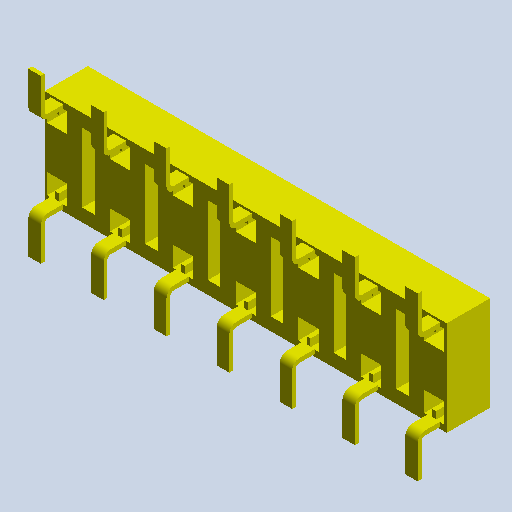
# Autodesk Inventor part: C-132-12-07-DV
Saved by Autodesk Inventor 2024.2 (Build 282272000, 272)
## iProperties
Category: PARTsolutions
Company: SAMTEC
Part Number: C-132-12-07-DV
Material: Generic
Catalog Web Link: www.cadenas.de
Description: C-132-Pins
Vendor: SAMTEC
Document SubType Name: Modeling
Designer: partserver
Manufacturer: SAMTEC
Mass: 0.0818982 g
Surface Area: 3.68105 cm^2
Volume: 0.0818982 cm^3
Density: 1 g/cm^3
Appearance: PSOLRGB-255-255-0
PSOL_IDENT_0: {$CADENAS_DATA\23d-libs\samtec\modelling\hle\parts\hle_pins.prj},176 {VTYP=3D},{NB=C-132-12-07-DV},{
PSOL_IDENT_1: LINA=C-132-12-07-DV},{NN=C-132},{DATE=08.04.2016 05:41:50},{GEOMDATE=08.04.2016 05:31:00},{VERSION=}
PSOL_IDENT_2: ,{LINEID=10},{WBVAR=POS,ESOPT},{WBNUMERIC=}  {NB=C-132-12-07-DV},{LINA=C-132-12-07-DV},{KT=DUMMY},{P
PSOL_IDENT_3: N=C-132-12-07-DV},{SERIES=HLE},{POSALG=  '02' , '-02' , '03' , '-03' , '04' , '-04' , '05' , '-05' ,
PSOL_IDENT_4: '06' , '-06' , '07' , '-07' , '08' , '-08' , '09' , '-09' , '10' , '-10' , '11' , '-11' , '12' , '-
PSOL_IDENT_5: 12' , '13' , '-13' , '14' , '-14' , '15' , '-15' , '16' , '-16' , '17' , '-17' , '18' , '-18' , '19'
PSOL_IDENT_6: , '-19' , '20' , '-20' , '21' , '-21' , '22' , '-22' , '23' , '-23' , '24' , '-24' , '25' , '-25' ,
PSOL_IDENT_7: '26' , '-26' , '27' , '-27' , '28' , '-28' , '29' , '-29' , '30' , '-30' , '31' , '-31' , '32' , '-
PSOL_IDENT_8: 32' , '33' , '-33' , '34' , '-34' , '35' , '-35' , '36' , '-36' , '37' , '-37' , '38' , '-38' , '39'
PSOL_IDENT_9: , '-39' , '40' , '-40'  , '41' , '-41' , '42' , '-42' , '43' , '-43' , '44' , '-44' , '45' , '-45'
PSOL_IDENT_10: , '46' , '-46' , '47' , '-47' , '48' , '-48' , '49' , '-49' , '50' , '-50'   , '51' , '-51' , '52' ,
PSOL_IDENT_11: '-52' , '53' , '-53' , '54' , '-54' , '55' , '-55' , '56' , '-56' , '57' , '-57' , '58' , '-58' , '
PSOL_IDENT_12: 59' , '-59' , '60' , '-60'  , '61' , '-61' , '62' , '-62' , '63' , '-63' , '64' , '-64' , '65' , '-6
PSOL_IDENT_13: 5' , '66' , '-66' , '67' , '-67' , '68' , '-68' , '69' , '-69' , '70' , '-70'  , '71' , '-71' , '72'
PSOL_IDENT_14: , '-72' , '73' , '-73' , '74' , '-74' , '75' , '-75'   },{POS=07},{LSALG=  '02' , '-02 - Surface Mo
PSOL_IDENT_15: unt'  },{LS=02},{ROPTALG=   'DV' , '-DV - Double Vertical'   },{ROPT=DV},{ESOPT=},{A=0.144},{B=0.138
PSOL_IDENT_16: },{L=0.700},{PINS=7},{H2=0.030},{W=0.2000},{PINH=0.025},{PINL=0.2590},{PINW=0.020},{PITCH=0.1000},{P
PSOL_IDENT_17: ITCH2=0.1000},{X=0.045},{ESOPTPN=}
NB: C-132-12-07-DV
NN: C-132
NT: Pins
NBSYN: $PN.
LINA: C-132-12-07-DV
CATALOG: Samtec
PN: C-132-12-07-DV
SERIES: HLE
POS: -07
LS: 02
ROPT: DV
ESOPT: Standard
A: 0.144
B: 0.138
L: 0.7
H2: 0.03
W: 0.2
PINH: 0.025
PINL: 0.259
PINW: 0.02
PITCH: 0.1
PITCH2: 0.1
X: 0.045
SUPPLIER: SAMTEC
ARTICLENO: C-132-12-07-DV
BOMINFO: C-132-12-07-DV
CREATOR: CADENAS GmbH
Title: C-132-12-07-DV
Author: Cadenas PARTsolutions
Comments: Pins
Autodesk Inventor part; units mm, degrees
sketch "Sketch_11" plane through (0, 2.5146, 0) normal (0, 1, 0) x (1, 0, 0)
  line L0 (-8.128, 1.9177) -> (-8.128, -1.9177)
  line L1 (-8.128, -1.9177) -> (8.128, -1.9177)
  line L2 (8.128, -1.9177) -> (8.128, 1.9177)
  line L3 (8.128, 1.9177) -> (-8.128, 1.9177)
  line L4 (7.2136, -0.8636) -> (7.2136, -1.6764)
  line L5 (7.2136, -1.6764) -> (7.5438, -1.6764)
  line L6 (7.5438, -1.6764) -> (7.5438, -1.3716)
  line L7 (7.5438, -1.3716) -> (7.6962, -1.3716)
  line L8 (7.6962, -1.3716) -> (7.6962, -1.6764)
  line L9 (7.6962, -1.6764) -> (8.0264, -1.6764)
  line L10 (8.0264, -1.6764) -> (8.0264, -0.8636)
  line L11 (8.0264, -0.8636) -> (7.2136, -0.8636)
  line L12 (7.2136, 0.8636) -> (8.0264, 0.8636)
  line L13 (8.0264, 0.8636) -> (8.0264, 1.6764)
  line L14 (8.0264, 1.6764) -> (7.6962, 1.6764)
  line L15 (7.6962, 1.6764) -> (7.6962, 1.3716)
  line L16 (7.6962, 1.3716) -> (7.5438, 1.3716)
  line L17 (7.5438, 1.3716) -> (7.5438, 1.6764)
  line L18 (7.5438, 1.6764) -> (7.2136, 1.6764)
  line L19 (7.2136, 1.6764) -> (7.2136, 0.8636)
  line L20 (6.096, 1.397) -> (6.096, -1.397)
  line L21 (6.096, -1.397) -> (6.604, -1.397)
  line L22 (6.604, -1.397) -> (6.604, 1.397)
  line L23 (6.604, 1.397) -> (6.096, 1.397)
  line L24 (4.6736, -0.8636) -> (4.6736, -1.6764)
  line L25 (4.6736, -1.6764) -> (5.0038, -1.6764)
  line L26 (5.0038, -1.6764) -> (5.0038, -1.3716)
  line L27 (5.0038, -1.3716) -> (5.1562, -1.3716)
  line L28 (5.1562, -1.3716) -> (5.1562, -1.6764)
  line L29 (5.1562, -1.6764) -> (5.4864, -1.6764)
  line L30 (5.4864, -1.6764) -> (5.4864, -0.8636)
  line L31 (5.4864, -0.8636) -> (4.6736, -0.8636)
  line L32 (4.6736, 0.8636) -> (5.4864, 0.8636)
  line L33 (5.4864, 0.8636) -> (5.4864, 1.6764)
  line L34 (5.4864, 1.6764) -> (5.1562, 1.6764)
  line L35 (5.1562, 1.6764) -> (5.1562, 1.3716)
  line L36 (5.1562, 1.3716) -> (5.0038, 1.3716)
  line L37 (5.0038, 1.3716) -> (5.0038, 1.6764)
  line L38 (5.0038, 1.6764) -> (4.6736, 1.6764)
  line L39 (4.6736, 1.6764) -> (4.6736, 0.8636)
  line L40 (3.556, 1.397) -> (3.556, -1.397)
  line L41 (3.556, -1.397) -> (4.064, -1.397)
  line L42 (4.064, -1.397) -> (4.064, 1.397)
  line L43 (4.064, 1.397) -> (3.556, 1.397)
  line L44 (2.1336, -0.8636) -> (2.1336, -1.6764)
  line L45 (2.1336, -1.6764) -> (2.4638, -1.6764)
  line L46 (2.4638, -1.6764) -> (2.4638, -1.3716)
  line L47 (2.4638, -1.3716) -> (2.6162, -1.3716)
  line L48 (2.6162, -1.3716) -> (2.6162, -1.6764)
  line L49 (2.6162, -1.6764) -> (2.9464, -1.6764)
  line L50 (2.9464, -1.6764) -> (2.9464, -0.8636)
  line L51 (2.9464, -0.8636) -> (2.1336, -0.8636)
  line L52 (2.1336, 0.8636) -> (2.9464, 0.8636)
  line L53 (2.9464, 0.8636) -> (2.9464, 1.6764)
  line L54 (2.9464, 1.6764) -> (2.6162, 1.6764)
  line L55 (2.6162, 1.6764) -> (2.6162, 1.3716)
  line L56 (2.6162, 1.3716) -> (2.4638, 1.3716)
  line L57 (2.4638, 1.3716) -> (2.4638, 1.6764)
  line L58 (2.4638, 1.6764) -> (2.1336, 1.6764)
  line L59 (2.1336, 1.6764) -> (2.1336, 0.8636)
  line L60 (1.016, 1.397) -> (1.016, -1.397)
  line L61 (1.016, -1.397) -> (1.524, -1.397)
  line L62 (1.524, -1.397) -> (1.524, 1.397)
  line L63 (1.524, 1.397) -> (1.016, 1.397)
  line L64 (-0.4064, -0.8636) -> (-0.4064, -1.6764)
  line L65 (-0.4064, -1.6764) -> (-0.0762, -1.6764)
  line L66 (-0.0762, -1.6764) -> (-0.0762, -1.3716)
  line L67 (-0.0762, -1.3716) -> (0.0762, -1.3716)
  line L68 (0.0762, -1.3716) -> (0.0762, -1.6764)
  line L69 (0.0762, -1.6764) -> (0.4064, -1.6764)
  line L70 (0.4064, -1.6764) -> (0.4064, -0.8636)
  line L71 (0.4064, -0.8636) -> (-0.4064, -0.8636)
  line L72 (-0.4064, 0.8636) -> (0.4064, 0.8636)
  line L73 (0.4064, 0.8636) -> (0.4064, 1.6764)
  line L74 (0.4064, 1.6764) -> (0.0762, 1.6764)
  line L75 (0.0762, 1.6764) -> (0.0762, 1.3716)
  line L76 (0.0762, 1.3716) -> (-0.0762, 1.3716)
  line L77 (-0.0762, 1.3716) -> (-0.0762, 1.6764)
  line L78 (-0.0762, 1.6764) -> (-0.4064, 1.6764)
  line L79 (-0.4064, 1.6764) -> (-0.4064, 0.8636)
  line L80 (-1.524, 1.397) -> (-1.524, -1.397)
  line L81 (-1.524, -1.397) -> (-1.016, -1.397)
  line L82 (-1.016, -1.397) -> (-1.016, 1.397)
  line L83 (-1.016, 1.397) -> (-1.524, 1.397)
  line L84 (-2.9464, -0.8636) -> (-2.9464, -1.6764)
  line L85 (-2.9464, -1.6764) -> (-2.6162, -1.6764)
  line L86 (-2.6162, -1.6764) -> (-2.6162, -1.3716)
  line L87 (-2.6162, -1.3716) -> (-2.4638, -1.3716)
  line L88 (-2.4638, -1.3716) -> (-2.4638, -1.6764)
  line L89 (-2.4638, -1.6764) -> (-2.1336, -1.6764)
  line L90 (-2.1336, -1.6764) -> (-2.1336, -0.8636)
  line L91 (-2.1336, -0.8636) -> (-2.9464, -0.8636)
  line L92 (-2.9464, 0.8636) -> (-2.1336, 0.8636)
  line L93 (-2.1336, 0.8636) -> (-2.1336, 1.6764)
  line L94 (-2.1336, 1.6764) -> (-2.4638, 1.6764)
  line L95 (-2.4638, 1.6764) -> (-2.4638, 1.3716)
  line L96 (-2.4638, 1.3716) -> (-2.6162, 1.3716)
  line L97 (-2.6162, 1.3716) -> (-2.6162, 1.6764)
  line L98 (-2.6162, 1.6764) -> (-2.9464, 1.6764)
  line L99 (-2.9464, 1.6764) -> (-2.9464, 0.8636)
  line L100 (-4.064, 1.397) -> (-4.064, -1.397)
  line L101 (-4.064, -1.397) -> (-3.556, -1.397)
  line L102 (-3.556, -1.397) -> (-3.556, 1.397)
  line L103 (-3.556, 1.397) -> (-4.064, 1.397)
  line L104 (-5.4864, -0.8636) -> (-5.4864, -1.6764)
  line L105 (-5.4864, -1.6764) -> (-5.1562, -1.6764)
  line L106 (-5.1562, -1.6764) -> (-5.1562, -1.3716)
  line L107 (-5.1562, -1.3716) -> (-5.0038, -1.3716)
  line L108 (-5.0038, -1.3716) -> (-5.0038, -1.6764)
  line L109 (-5.0038, -1.6764) -> (-4.6736, -1.6764)
  line L110 (-4.6736, -1.6764) -> (-4.6736, -0.8636)
  line L111 (-4.6736, -0.8636) -> (-5.4864, -0.8636)
  line L112 (-5.4864, 0.8636) -> (-4.6736, 0.8636)
  line L113 (-4.6736, 0.8636) -> (-4.6736, 1.6764)
  line L114 (-4.6736, 1.6764) -> (-5.0038, 1.6764)
  line L115 (-5.0038, 1.6764) -> (-5.0038, 1.3716)
  line L116 (-5.0038, 1.3716) -> (-5.1562, 1.3716)
  line L117 (-5.1562, 1.3716) -> (-5.1562, 1.6764)
  line L118 (-5.1562, 1.6764) -> (-5.4864, 1.6764)
  line L119 (-5.4864, 1.6764) -> (-5.4864, 0.8636)
  line L120 (-6.604, 1.397) -> (-6.604, -1.397)
  line L121 (-6.604, -1.397) -> (-6.096, -1.397)
  line L122 (-6.096, -1.397) -> (-6.096, 1.397)
  line L123 (-6.096, 1.397) -> (-6.604, 1.397)
  line L124 (-8.0264, -0.8636) -> (-8.0264, -1.6764)
  line L125 (-8.0264, -1.6764) -> (-7.6962, -1.6764)
  line L126 (-7.6962, -1.6764) -> (-7.6962, -1.3716)
  line L127 (-7.6962, -1.3716) -> (-7.5438, -1.3716)
  line L128 (-7.5438, -1.3716) -> (-7.5438, -1.6764)
  line L129 (-7.5438, -1.6764) -> (-7.2136, -1.6764)
  line L130 (-7.2136, -1.6764) -> (-7.2136, -0.8636)
  line L131 (-7.2136, -0.8636) -> (-8.0264, -0.8636)
  line L132 (-8.0264, 0.8636) -> (-7.2136, 0.8636)
  line L133 (-7.2136, 0.8636) -> (-7.2136, 1.6764)
  line L134 (-7.2136, 1.6764) -> (-7.5438, 1.6764)
  line L135 (-7.5438, 1.6764) -> (-7.5438, 1.3716)
  line L136 (-7.5438, 1.3716) -> (-7.6962, 1.3716)
  line L137 (-7.6962, 1.3716) -> (-7.6962, 1.6764)
  line L138 (-7.6962, 1.6764) -> (-8.0264, 1.6764)
  line L139 (-8.0264, 1.6764) -> (-8.0264, 0.8636)
  constraints: 280 end point
extrude "Extrusion1" add sketch "Sketch_11" against normal blind 1.7526
sketch "Sketch_12" plane through (0, 0, 0) normal (1, 0, 0) x (0, 1, 0)
  line L0 (-0.1524, 3.2893) -> (-0.1524, 1.9558)
  arc A0 (-0.1524, 1.9558) -> (0.1524, 1.651) centre (0.1524, 1.9558) ccw
  line L1 (0.1524, 1.651) -> (0.762, 1.651)
  line L2 (0.762, 1.651) -> (0.762, 1.8288)
  line L3 (0.762, 1.8288) -> (0.127, 1.8288)
  arc A1 (0, 1.9558) -> (0.127, 1.8288) centre (0.127, 1.9558) ccw
  line L4 (0, 1.9558) -> (0, 3.2893)
  line L5 (0, 3.2893) -> (-0.1524, 3.2893)
  constraints: 12 end point, 4 point on circle, 2 centre point
extrude "Extrusion2" add sketch "Sketch_12" along normal mid plane 16.256
sketch "Sketch_13" plane through (0, 0, 0) normal (1, 0, 0) x (0, 1, 0)
  arc A0 (0.1524, -1.651) -> (-0.1524, -1.9558) centre (0.1524, -1.9558) ccw
  line L0 (-0.1524, -1.9558) -> (-0.1524, -3.2893)
  line L1 (-0.1524, -3.2893) -> (0, -3.2893)
  line L2 (0, -3.2893) -> (0, -1.9558)
  arc A1 (0.127, -1.8288) -> (0, -1.9558) centre (0.127, -1.9558) ccw
  line L3 (0.127, -1.8288) -> (0.762, -1.8288)
  line L4 (0.762, -1.8288) -> (0.762, -1.651)
  line L5 (0.762, -1.651) -> (0.1524, -1.651)
  constraints: 12 end point, 4 point on circle, 2 centre point
extrude "Extrusion3" add sketch "Sketch_13" along normal mid plane 16.256
sketch "Sketch_5" plane through (0, 0, 0) normal (0, 0, 1) x (1, 0, 0)
  line L0 (-10.414, -3.556) -> (9.906, -3.556)
  line L1 (9.906, -3.556) -> (9.906, 0.762)
  line L2 (9.906, 0.762) -> (7.874, 0.762)
  line L3 (7.874, 0.762) -> (7.874, -3.048)
  line L4 (7.874, -3.048) -> (7.366, -3.048)
  line L5 (7.366, -3.048) -> (7.366, 0.762)
  line L6 (7.366, 0.762) -> (5.334, 0.762)
  line L7 (5.334, 0.762) -> (5.334, -3.048)
  line L8 (5.334, -3.048) -> (4.826, -3.048)
  line L9 (4.826, -3.048) -> (4.826, 0.762)
  line L10 (4.826, 0.762) -> (2.794, 0.762)
  line L11 (2.794, 0.762) -> (2.794, -3.048)
  line L12 (2.794, -3.048) -> (2.286, -3.048)
  line L13 (2.286, -3.048) -> (2.286, 0.762)
  line L14 (2.286, 0.762) -> (0.254, 0.762)
  line L15 (0.254, 0.762) -> (0.254, -3.048)
  line L16 (0.254, -3.048) -> (-0.254, -3.048)
  line L17 (-0.254, -3.048) -> (-0.254, 0.762)
  line L18 (-0.254, 0.762) -> (-2.286, 0.762)
  line L19 (-2.286, 0.762) -> (-2.286, -3.048)
  line L20 (-2.286, -3.048) -> (-2.794, -3.048)
  line L21 (-2.794, -3.048) -> (-2.794, 0.762)
  line L22 (-2.794, 0.762) -> (-4.826, 0.762)
  line L23 (-4.826, 0.762) -> (-4.826, -3.048)
  line L24 (-4.826, -3.048) -> (-5.334, -3.048)
  line L25 (-5.334, -3.048) -> (-5.334, 0.762)
  line L26 (-5.334, 0.762) -> (-7.366, 0.762)
  line L27 (-7.366, 0.762) -> (-7.366, -3.048)
  line L28 (-7.366, -3.048) -> (-7.874, -3.048)
  line L29 (-7.874, -3.048) -> (-7.874, 0.762)
  line L30 (-7.874, 0.762) -> (-10.414, 0.762)
  line L31 (-10.414, 0.762) -> (-10.414, -3.556)
  constraints: 64 end point
extrude "Extrusion4" cut sketch "Sketch_5" along normal mid plane 10.16
ref_plane "pins_to_socket_XY" through (0, 0, 0) normal (0, 1, 0) x (1, 0, 0)
ref_plane "pins_to_socket_YZ" through (0, 0, 0) normal (1, 0, 0) x (0, 0, -1)
ref_plane "pins_to_socket_ZX" through (0, 0, 0) normal (0, 0, -1) x (0, 1, 0)
body "Solid1"
